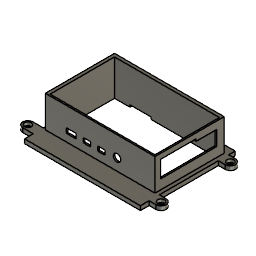
Pi Cover and Stand (Autodesk Fusion 360 design; units mm, degrees)
Autodesk Fusion 360 part; units mm, degrees
sketch "Sketch2" plane through (0, 0, 0) normal (0, 0, 1) x (-1, 0, 0)
  line L0 (54.875, -44.875) -> (-54.875, -44.875)
  line L1 (-54.875, -44.875) -> (-54.875, 44.875)
  line L2 (-54.875, 44.875) -> (54.875, 44.875)
  line L3 (54.875, 44.875) -> (54.875, -44.875)
  point P0 (0, -44.875)
  point P1 (-54.875, 0)
  dimension "d76" = 109.75
  dimension "d77" = 89.75
  constraint horizontal L0
  constraint vertical L1
  constraint horizontal L2
  constraint vertical L3
  constraint midpoint L0 P0
  constraint midpoint L1 P1
  constraint vertical origin P0
  constraint horizontal origin P1
  measures "d76" distance of L0.start L0.end
  measures "d77" distance of L0.end L1.end
extrude "Extrude2" add sketch "Sketch2" along normal mid plane 4
sketch "Sketch3" plane through (0, 0, 2) normal (0, 0, 1) x (-1, 0, 0)
  line L0 (54.875, 44.875) -> (-54.875, 44.875)
  line L1 (-54.875, 44.875) -> (-54.875, -44.875)
  line L2 (-54.875, -44.875) -> (54.875, -44.875)
  line L3 (54.875, -44.875) -> (54.875, 44.875)
  line L4 (39.375, -31.875) -> (-45.625, -31.875) construction
  line L5 (-45.625, -31.875) -> (-45.625, 24.125) construction
  line L6 (-45.625, 24.125) -> (39.375, 24.125) construction
  line L7 (39.375, 24.125) -> (39.375, -31.875) construction
  line L8 (49.375, -34.875) -> (-49.925, -34.875)
  line L9 (-49.925, -34.875) -> (-49.925, 26.125)
  line L10 (-49.925, 26.125) -> (49.375, 26.125)
  line L11 (49.375, 26.125) -> (49.375, -34.875)
  point P0 (35.875, -28.375)
  point P1 (35.875, 20.625)
  point P2 (-22.125, -28.375)
  point P3 (-22.125, 20.625)
  dimension "d11" = 85
  dimension "d12" = 56
  dimension "d13" = 13
  dimension "d14" = 15.5
  dimension "d15" = 3.5
  dimension "d16" = 3.5
  dimension "d17" = 3.5
  dimension "d18" = 3.5
  dimension "d19" = 58
  dimension "d20" = 58
  dimension "d21" = 2
  dimension "d22" = 10
  dimension "d23" = 4.3
  dimension "d24" = 3
  constraint horizontal L4
  constraint vertical L5
  constraint horizontal L6
  constraint vertical L7
  constraint horizontal P0 P2
  constraint horizontal P1 P3
  constraint horizontal L8
  constraint vertical L9
  constraint horizontal L10
  constraint vertical L11
  measures "d11" distance of L4.start L4.end
  measures "d12" distance of L4.end L5.end
  measures "d13" distance of L2 L4
  measures "d14" distance of L3 L7
  measures "d15" distance of L4 P0
  measures "d16" distance of L7 P0
  measures "d17" distance of L6 P1
  measures "d18" distance of L7 P1
  measures "d19" distance of P0 P2
  measures "d20" distance of P1 P3
  measures "d21" distance of L5.end L10
  measures "d22" distance of L7 L11
  measures "d23" distance of L5 L9
  measures "d24" distance of L4 L8
extrude "Extrude3" cut sketch "Sketch3" against normal through all contours L8 L9 L10 L11
sketch "Sketch4" plane through (0, 0, 2) normal (0, 0, 1) x (-1, 0, 0)
  line L0 (49.375, 26.125) -> (49.375, -34.875)
  line L1 (49.375, -34.875) -> (-49.925, -34.875)
  line L2 (-49.925, -34.875) -> (-49.925, 26.125)
  line L3 (-49.925, 26.125) -> (49.375, 26.125)
  line L4 (54.875, 44.875) -> (-54.875, 44.875)
  line L5 (-54.875, 44.875) -> (-54.875, -44.875)
  line L6 (-54.875, -44.875) -> (54.875, -44.875)
  line L7 (54.875, -44.875) -> (54.875, 44.875)
  line L8 (49.375, -34.875) -> (-49.925, -34.875)
  line L9 (-49.925, -34.875) -> (-49.925, 26.125)
  line L10 (-49.925, 26.125) -> (49.375, 26.125)
  line L11 (49.375, 26.125) -> (49.375, -34.875)
  line L12 (52.375, -37.875) -> (-51.425, -37.875)
  line L13 (-51.425, -37.875) -> (-51.425, 27.625)
  line L14 (-51.425, 27.625) -> (52.375, 27.625)
  line L15 (52.375, 27.625) -> (52.375, -37.875)
  dimension "d26" = 1.5
  dimension "d27" = 1.5
  dimension "d28" = 3
  dimension "d29" = 3
  constraint horizontal L8
  constraint vertical L9
  constraint horizontal L10
  constraint vertical L11
  constraint coincident L2.end L3.start
  constraint coincident L0.end L1.start
  constraint horizontal L12
  constraint vertical L13
  constraint horizontal L14
  constraint vertical L15
  measures "d26" distance of L10 L14
  measures "d27" distance of L9 L13
  measures "d28" distance of L8 L12
  measures "d29" distance of L11 L15
extrude "Extrude4" add sketch "Sketch4" along normal blind 30 contours L12 L13 L14 L15
sketch "Sketch5" plane through (0, -27.625, 0) normal (0, -1, 0) x (1, 0, 0)
  line L0 (-52.375, 2) -> (51.425, 2)
  line L1 (51.425, 2) -> (51.425, 32)
  line L2 (51.425, 32) -> (-52.375, 32)
  line L3 (-52.375, 32) -> (-52.375, 2)
  line L4 (-32.475, 13.6) -> (-23.305, 13.6)
  line L5 (-23.305, 13.6) -> (-23.305, 9.15)
  line L6 (-23.305, 9.15) -> (-32.475, 9.15)
  line L7 (-32.475, 9.15) -> (-32.475, 13.6)
  line L8 (-16.405, 13.6) -> (-9.545, 13.6)
  line L9 (-9.545, 13.6) -> (-9.545, 9.35)
  line L10 (-9.545, 9.35) -> (-16.405, 9.35)
  line L11 (-16.405, 9.35) -> (-16.405, 13.6)
  line L12 (4.065, 9.35) -> (-2.795, 9.35)
  line L13 (-2.795, 13.6) -> (4.065, 13.6)
  line L14 (4.065, 13.6) -> (4.065, 9.35)
  line L15 (-2.795, 9.35) -> (-2.795, 13.6)
  circle A0 centre (15.515, 13) radius 3.5
  line L16 (49.925, 2) -> (-49.375, 2)
  point P0 (-39.375, 2)
  point P1 (12.015, 13)
  dimension "d32" = 7.15
  dimension "d33" = 6.9
  dimension "d34" = 9.17
  dimension "d35" = 4.45
  dimension "d36" = 6.86
  dimension "d37" = 4.25
  dimension "d38" = 6.9
  dimension "d39" = 6.86
  dimension "d40" = 4.25
  dimension "d41" = 6.75
  dimension "d42" = 7
  dimension "d74" = 11
  dimension "d75" = 7.95
  constraint horizontal L4
  constraint vertical L5
  constraint horizontal L6
  constraint vertical L7
  constraint horizontal L8
  constraint vertical L9
  constraint horizontal L10
  constraint vertical L11
  constraint horizontal L4.end L8.start
  constraint horizontal L13
  constraint vertical L14
  constraint horizontal L12
  constraint vertical L15
  constraint horizontal L8.end L13.start
  constraint coincident A0 P1
  constraint horizontal A0.centre P1
  measures "d32" distance of L0 L6
  measures "d33" horizontal distance of L6.end P0
  measures "d34" distance of L4.start L4.end
  measures "d35" distance of L4.end L5.end
  measures "d36" distance of L8.start L8.end
  measures "d37" distance of L8.end L9.end
  measures "d38" distance of L5 L11
  measures "d39" distance of L13.start L13.end
  measures "d40" distance of L13.end L12.start
  measures "d41" distance of L9 L15
  measures "d42" diameter of A0
  measures "d74" distance of A0.centre L16
  measures "d75" horizontal distance of L13.end P1
extrude "Extrude5" cut sketch "Sketch5" against normal up to surface (1.5 mm away) contours L4 L5 L6 L7 | L8 L9 L10 L11 | L12 L13 L14 L15 | A0
fillet "Fillet1" radius 0.5 12 edges at (-32.475, -26.875, 13.6) (-32.475, -26.875, 9.15) (-23.305, -26.875, 9.15) (-23.305, -26.875, 13.6) (-9.545, -26.875, 13.6) (4.065, -26.875, 13.6) (-2.795, -26.875, 13.6) (-16.405, -26.875, 13.6) (-9.545, -26.875, 9.35) (4.065, -26.875, 9.35) (-2.795, -26.875, 9.35) (-16.405, -26.875, 9.35)
sketch "Sketch6" plane through (51.425, 0, 0) normal (1, 0, 0) x (0, 1, 0)
  line L0 (-27.625, 2) -> (37.875, 2)
  line L1 (37.875, 2) -> (37.875, 32)
  line L2 (37.875, 32) -> (-27.625, 32)
  line L3 (-27.625, 32) -> (-27.625, 2)
  line L4 (-22.225, 27) -> (-4.225, 27)
  line L5 (-4.225, 11) -> (-22.225, 11)
  line L6 (-22.225, 11) -> (-22.225, 27)
  line L7 (34.875, 2) -> (-26.125, 2)
  line L8 (-4.225, 27) -> (11.275, 27)
  line L9 (11.275, 11) -> (-4.225, 11)
  line L10 (11.275, 27) -> (11.275, 25)
  line L11 (11.275, 25) -> (30.775, 25)
  line L12 (30.775, 25) -> (30.775, 11)
  line L13 (30.775, 11) -> (11.275, 11)
  point P0 (-24.125, 2)
  dimension "d50" = 16
  dimension "d51" = 9
  dimension "d53" = 16
  dimension "d56" = 14
  dimension "d72" = 5.4
  dimension "d95" = 33.5
  dimension "d96" = 19.5
  constraint horizontal L4
  constraint horizontal L5
  constraint vertical L6
  constraint horizontal L8
  constraint vertical L10
  constraint horizontal L9
  constraint horizontal L5.start L9.end
  constraint horizontal L11
  constraint vertical L12
  constraint horizontal L13
  constraint horizontal L9.start L13.end
  constraint coincident L4.end L8.start
  constraint coincident L5.start L9.end
  constraint coincident L9.start L13.end
  measures "d50" distance of L4.start L5.end
  measures "d51" distance of L5 L7
  measures "d53" distance of L4.end L5.start
  measures "d56" distance of L11.end L12.end
  measures "d72" distance of L3 L6
  measures "d95" distance of L4.start L8.end
  measures "d96" distance of L10.end L11.end
extrude "Extrude6" cut sketch "Sketch6" against normal up to surface (1.5 mm away) contours L4 L5 L6 L8 L9 L10 L11 L12 L13
sketch "Sketch9" plane through (0, 0, -2) normal (0, 0, -1) x (1, 0, 0)
  line L0 (-49.375, -34.875) -> (-49.375, 26.125)
  line L1 (-49.375, 26.125) -> (49.925, 26.125)
  line L2 (49.925, 26.125) -> (49.925, -34.875)
  line L3 (49.925, -34.875) -> (-49.375, -34.875)
  line L4 (54.875, 44.875) -> (-54.875, 44.875)
  line L5 (-54.875, 44.875) -> (-54.875, -44.875)
  line L6 (-54.875, -44.875) -> (54.875, -44.875)
  line L7 (54.875, -44.875) -> (54.875, 44.875)
  line L8 (61.325, 36.6) -> (54.875, 36.6)
  line L9 (61.325, 26.85) -> (54.875, 26.85)
  line L10 (61.325, -28.95) -> (54.875, -28.95)
  line L11 (61.325, -38.7) -> (54.875, -38.7)
  line L12 (-64.805, -38.7) -> (-54.875, -38.7)
  line L13 (-64.805, -28.95) -> (-54.875, -28.95)
  line L14 (-64.805, 26.85) -> (-54.875, 26.85)
  line L15 (-64.805, 36.6) -> (-54.875, 36.6)
  arc A0 (-64.805, -28.95) -> (-64.805, -38.7) centre (-64.805, -33.825) ccw
  arc A1 (61.325, -38.7) -> (61.325, -28.95) centre (61.325, -33.825) ccw
  arc A2 (61.325, 26.85) -> (61.325, 36.6) centre (61.325, 31.725) ccw
  arc A3 (-64.805, 36.6) -> (-64.805, 26.85) centre (-64.805, 31.725) ccw
  dimension "d78" = 9.75
  dimension "d79" = 6.45
  dimension "d80" = 126.13
  dimension "d81" = 65.55
  dimension "d82" = 13.15
  constraint coincident L7 L8.end
  constraint tangent L8 A2
  constraint tangent L9 A2
  constraint perpendicular L7 L9
  constraint parallel L8 L10
  constraint coincident L11.start A1
  constraint coincident L7 L11.end
  constraint coincident L12.start A0
  constraint coincident L5 L12.end
  constraint coincident L5 L13.end
  constraint tangent L13 A0
  constraint coincident L5 L14.end
  constraint coincident L5 L15.end
  constraint tangent L15 A3
  constraint tangent L14 A3
  constraint horizontal L15
  constraint horizontal L14
  constraint horizontal L8
  constraint horizontal L11
  constraint horizontal L13
  constraint horizontal L12
  constraint equal A1 A2
  constraint equal A2 A3
  constraint equal A0 A2
  constraint vertical A0.centre A3.centre
  constraint vertical A2.centre A1.centre
  constraint horizontal A1.centre A0.centre
  constraint horizontal A2.centre A3.centre
  constraint coincident L12 A0.end
  constraint coincident L11 A1.start
  constraint tangent L12 A0
  constraint tangent L10 A1
  constraint tangent L11 A1
  measures "d78" diameter of A2
  measures "d79" distance of L7 A2.centre
  measures "d80" horizontal distance of A2.centre A3.centre
  measures "d81" distance of A0.centre A3.centre
  measures "d82" distance of L4 A2.centre
extrude "Extrude8" add sketch "Sketch9" against normal up to surface (4 mm away) contours L7 L8 L9 A2 | L5 L14 L15 A3 | L7 L10 L11 A1 | L5 L12 L13 A0
sketch "Sketch10" plane through (0, 0, 2) normal (0, 0, 1) x (-1, 0, 0)
  line L0 (52.375, 27.625) -> (52.375, -37.875)
  line L1 (52.375, -37.875) -> (-51.425, -37.875)
  line L2 (-51.425, -37.875) -> (-51.425, 27.625)
  line L3 (-51.425, 27.625) -> (52.375, 27.625)
  line L4 (54.875, 44.875) -> (-54.875, 44.875)
  line L5 (-54.875, 44.875) -> (-54.875, 36.6)
  line L6 (-54.875, 36.6) -> (-61.325, 36.6)
  arc A0 (-61.325, 36.6) -> (-61.325, 26.85) centre (-61.325, 31.725) ccw
  line L7 (-61.325, 26.85) -> (-54.875, 26.85)
  line L8 (-54.875, 26.85) -> (-54.875, -28.95)
  line L9 (-54.875, -28.95) -> (-61.325, -28.95)
  arc A1 (-61.325, -28.95) -> (-61.325, -38.7) centre (-61.325, -33.825) ccw
  line L10 (-61.325, -38.7) -> (-54.875, -38.7)
  line L11 (-54.875, -38.7) -> (-54.875, -44.875)
  line L12 (-54.875, -44.875) -> (54.875, -44.875)
  line L13 (54.875, -44.875) -> (54.875, -38.7)
  line L14 (54.875, -38.7) -> (64.805, -38.7)
  arc A2 (64.805, -38.7) -> (64.805, -28.95) centre (64.805, -33.825) ccw
  line L15 (64.805, -28.95) -> (54.875, -28.95)
  line L16 (54.875, -28.95) -> (54.875, 26.85)
  line L17 (54.875, 26.85) -> (64.805, 26.85)
  arc A3 (64.805, 26.85) -> (64.805, 36.6) centre (64.805, 31.725) ccw
  line L18 (64.805, 36.6) -> (54.875, 36.6)
  line L19 (54.875, 36.6) -> (54.875, 44.875)
  point P0 (64.805, -33.825)
  point P1 (64.805, 31.725)
  point P2 (-61.325, -33.825)
  point P3 (-61.325, 31.725)
  constraint coincident P0 A2.centre
  constraint coincident P1 A3.centre
  constraint coincident P2 A1.centre
  constraint coincident P3 A0.centre
hole "Hole3" at (-64.805, 33.825, 2) at (61.325, 33.825, 2) at (61.325, -31.725, 2) at (-64.805, -31.725, 2) direction (0, 0, -1) diameter 3.4 depth 12 tip angle 118 counterbore diameter 6.5 counterbore depth 3
sketch "Sketch11" plane through (0, 44.875, 0) normal (0, 1, 0) x (-1, 0, 0)
  line L0 (54.875, -2) -> (54.875, 2)
  line L1 (54.875, 2) -> (-54.875, 2)
  line L2 (-54.875, 2) -> (-54.875, -2)
  line L3 (-54.875, -2) -> (54.875, -2)
  line L4 (14.875, 0) -> (34.875, 0)
  line L5 (34.875, 0) -> (34.875, -2)
  line L6 (34.875, -2) -> (14.875, -2)
  line L7 (14.875, -2) -> (14.875, 0)
  dimension "d90" = 20
  dimension "d91" = 20
  dimension "d92" = 2
  constraint horizontal L4
  constraint vertical L5
  constraint horizontal L6
  constraint vertical L7
  constraint coincident L3 L5.end
  measures "d90" distance of L0 L5
  measures "d91" distance of L4.start L4.end
  measures "d92" distance of L4.start L6.end
extrude "Extrude9" cut sketch "Sketch11" against normal up to surface (10 mm away) contours L3 L4 L5 L6 L7
equation "d16 = d15"
equation "d17 = d15"
equation "d18 = d15"
equation "d29 = d28"
equation "d30 = 25.5 mm + 4.5 mm"
equation "d32 = 4.4 mm + 4.25 mm - 1.5 mm"
equation "d33 = 6.7 mm - 0.25 mm + 3 mm - 2.15 mm - 0.4 mm"
equation "d72 = 6.25 mm - 1 mm + 1.15 mm - 1 mm"
equation "d74 = 8.5 mm + 4 mm - 1.5 mm"
equation "d76 = 110 mm - 0.25 mm"
equation "d77 = 90 mm - 0.25 mm"
equation "d78 = 10 mm - 0.25 mm"
equation "d79 = 6.325 mm + ( 0.25 / 2 ) * 1 mm"
equation "d82 = 13.025 mm + ( 0.25 / 2 ) * 1 mm"
